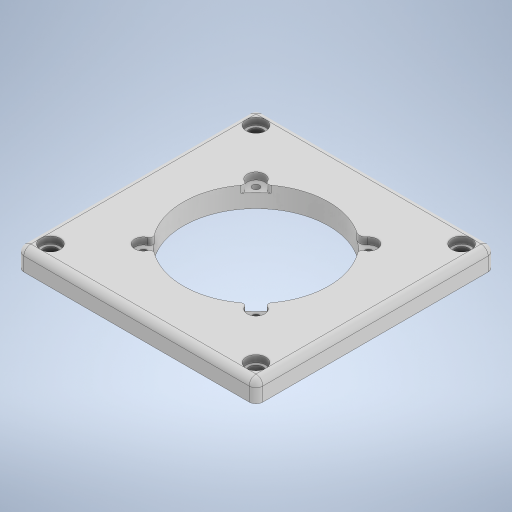
# Autodesk Inventor part: joystickBOXtop
Saved by Autodesk Inventor 2023 (Build 270158000, 158)
## iProperties
Created: 2023-09-26
Part Number: joystickBOXtop
Material: Generic
Document SubType Name: Modeling
Designer: Nikita
Density: 1 g/cm^3
Appearance: Default
Author: Nikita
Autodesk Inventor part; units mm, degrees
ref_plane "YZ Plane" through (0, 0, 0) normal (1, 0, 0) x (0, 1, 0)
ref_plane "XZ Plane" through (0, 0, 0) normal (0, 1, 0) x (-1, 0, 0)
ref_plane "XY Plane" through (0, 0, 0) normal (0, 0, 1) x (1, 0, 0)
sketch "Sketch1" plane through (0, 0, 0) normal (0, 1, 0) x (-1, 0, 0)
  line L0 (0, 0) -> (69, 0)
  line L1 (69, 0) -> (69, -69)
  line L2 (69, -69) -> (0, -69)
  line L3 (0, -69) -> (0, 0)
  dimension "d0" = 69
  dimension "d1" = 69
  constraints: 8 end point, 3 perpendicular, 1 horizontal
  measures "d0" distance of L0.start L0.end
  measures "d1" distance of L0.end L1.end
extrude "Extrusion1" add sketch "Sketch1" along normal blind 6
sketch "Sketch2" plane through (0, 6, 0) normal (0, 1, 0) x (1, 0, 0)
  line L0 (0, 0) -> (0, 69) construction
  line L1 (0, 69) -> (-69, 69) construction
  line L2 (0, 0) -> (-69, 69) construction
  line L3 (-69, 69) -> (-69, 0) construction
  line L4 (-69, 0) -> (0, 69) construction
  circle A0 centre (-34.5, 34.5) radius 21
  dimension "d4" = 42
  constraints: 6 end point, 2 perpendicular, 1 centre point, 1 midpoint
  measures "d4" diameter of A0
extrude "Extrusion2" cut sketch "Sketch2" against normal blind 6
fillet "Fillet1" radius 2 1 edges at (-34.5, 6, 0)
fillet "Fillet2" radius 2 3 edges at (0, 6, -35.5) (0, 5.4142, -0.5858) (0, 2, 0)
fillet "Fillet3" radius 2 3 edges at (-0.5858, 5.4142, -69) (0, 2, -69) (-35.5, 6, -69)
fillet "Fillet4" radius 2 5 edges at (-69, 5.4142, -0.5858) (-69, 2, 0) (-69, 5.4142, -68.4142) (-69, 2, -69) (-69, 6, -34.5)
sketch "Sketch3" plane through (0, 6, 0) normal (0, 1, 0) x (1, 0, 0)
  line L0 (-67, 69) -> (-67, 67) construction
  line L1 (-2, 2) -> (-67, 2) construction
  line L2 (-67, 67) -> (-2, 2) construction
  line L3 (-67, 67) -> (-2, 67) construction
  line L4 (-67, 2) -> (-67, 67) construction
  line L5 (-2, 67) -> (-67, 2) construction
  line L6 (-34.5, 34.5) -> (-18.2507, 18.2507) construction
  line L7 (-18.2507, 18.2507) -> (-18.2493, 50.7507) construction
  line L8 (-18.2493, 50.7507) -> (-50.7521, 50.7521) construction
  line L9 (-50.7521, 50.7521) -> (-50.7521, 18.2479) construction
  line L10 (-18.2507, 18.2507) -> (-50.7521, 18.2479) construction
  circle A0 centre (-34.5, 34.5) radius 20.5 construction
  circle A1 centre (-18.2493, 50.7507) radius 1
  point P0 (0, 0)
  dimension "d11" = 22.98
  dimension "d12" = 32.5
  dimension "d13" = 41
  dimension "d14" = 2
  constraints: 14 end point, 4 point on line, 2 centre point, 2 coincident, 1 midpoint, 1 perpendicular, 1 vertical
  measures "d11" distance of L6.start L6.end
  measures "d12" distance of L6.end L7.end
  measures "d13" diameter of A0
  measures "d14" diameter of A1
extrude "Extrusion3" cut sketch "Sketch3" against normal blind 10
pattern_circular "Circular Pattern1" count 4 over 360 about axis through (-34.5, 6, -34.5) along (0, -1, 0) of "Extrusion3"
sketch "Sketch5" plane through (0, 6, 0) normal (0, 1, 0) x (1, 0, 0)
  circle A0 centre (-18.2493, 50.7507) radius 2.5
  circle A1 centre (-18.2493, 50.7507) radius 1 projected
  point P0 (0, 0)
  dimension "d20" = 5
  constraints: 1 centre point, 1 coincident
  measures "d20" diameter of A0
extrude "Extrusion4" cut sketch "Sketch5" against normal blind 2 contours A0 | A1
pattern_circular "Circular Pattern2" count 4 over 360 about axis through (-34.5, 6, -34.5) along (0, -1, 0) of "Extrusion4"
fillet "Fillet5" radius 1 1 edges at (-48.2842, 5, -50.3429)
fillet "Fillet6" radius 1 1 edges at (-50.3429, 5, -48.2842)
fillet "Fillet7" radius 1 1 edges at (-50.3429, 5, -20.7158)
fillet "Fillet8" radius 1 1 edges at (-48.2842, 5, -18.6571)
fillet "Fillet9" radius 1 1 edges at (-20.7158, 5, -18.6571)
fillet "Fillet10" radius 1 1 edges at (-18.6571, 5, -20.7158)
fillet "Fillet11" radius 1 1 edges at (-18.6571, 5, -48.2842)
sketch "Sketch6" plane through (0, 6, 0) normal (0, 1, 0) x (1, 0, 0)
  line L0 (-2, 67) -> (-2, 2) projected
  arc A0 (-2, 0) -> (0, 2) centre (-2, 2) ccw projected
  line L1 (0, 2) -> (-2, 2) projected
  line L2 (0, 0) -> (-2, 2)
  line L3 (-0.5858, 0.5858) -> (-4.8284, 4.8284) construction
  circle A1 centre (-4.8284, 4.8284) radius 2
  dimension "d52" = 6
  dimension "d53" = 4
  constraints: 4 end point, 2 point on line, 1 centre point, 1 coincident, 1 point on circle
  measures "d52" distance of L3.start L3.end
  measures "d53" diameter of A1
extrude "Extrusion5" cut sketch "Sketch6" against normal blind 18.75 contours A1
pattern_linear "Rectangular Pattern1" count 2 spacing 59.343 along (0, 0, -1) count 2 spacing 59.343 along (-1, 0, 0) of "Extrusion5"
sketch "Sketch8" plane through (0, 6, 0) normal (0, 1, 0) x (1, 0, 0)
  line L0 (-2, 2) -> (-67, 2) projected
  circle A0 centre (-4.8284, 4.8284) radius 2 construction
  line L1 (-4.8284, 4.8284) -> (-2, 2) construction
  circle A1 centre (-4.8284, 4.8284) radius 2.8284 construction
  circle A2 centre (-4.8284, 4.8284) radius 2.8284
  circle A3 centre (-4.8284, 4.8284) radius 2
  point P0 (0, 0)
  point P1 (-4.1213, 4.1213)
  constraints: 3 centre point, 3 coincident, 2 concentric, 2 end point, 1 tangent
extrude "Extrusion6" cut sketch "Sketch8" against normal blind 2 contours A2 | A3
pattern_linear "Rectangular Pattern2" count 2 spacing 59.343 along (-1, 0, 0) count 2 spacing 59.343 along (0, 0, -1) of "Extrusion6"
fillet "Fillet12" radius 2 1 edges at (-20.7158, 5, -50.3429)
equation "\"d0\" = d1"
body "Solid1"
